Autodesk Fusion 360 part; units mm, degrees
(part 4 of 5)
  line L2596 (100.9284, -91.6876) -> (100.9149, -91.7012)
  line L2597 (100.9149, -91.7012) -> (100.9053, -91.7031)
  line L2598 (100.9053, -91.7031) -> (98.5241, -91.7031)
  line L2599 (98.5241, -91.7031) -> (98.5145, -91.7012)
  line L2600 (98.5145, -91.7012) -> (98.501, -91.6876)
  line L2601 (98.501, -91.6876) -> (98.4991, -91.6781)
  line L2602 (98.4991, -91.6781) -> (98.4991, -89.6195)
  line L2603 (98.4991, -89.6195) -> (96.1428, -89.6195)
  line L2604 (96.1428, -89.6195) -> (96.1333, -89.6176)
  line L2605 (96.1333, -89.6176) -> (96.1197, -89.6041)
  line L2606 (96.1197, -89.6041) -> (96.1178, -89.5945)
  line L2607 (96.1178, -89.5945) -> (96.1178, -86.3203)
  line L2608 (96.1178, -86.3203) -> (96.1197, -86.3107)
  line L2609 (96.1197, -86.3107) -> (96.1333, -86.2972)
  line L2610 (96.1333, -86.2972) -> (96.1428, -86.2953)
  line L2611 (96.1428, -86.2953) -> (98.4991, -86.2953)
  line L2612 (98.4991, -86.2953) -> (98.4991, -83.3437)
  line L2613 (98.4991, -83.3437) -> (98.501, -83.3341)
  line L2614 (98.501, -83.3341) -> (98.5145, -83.3206)
  line L2615 (98.5145, -83.3206) -> (98.5241, -83.3187)
  line L2616 (98.5241, -83.3187) -> (112.2163, -83.3187)
  line L2617 (112.2163, -83.3187) -> (112.2258, -83.3206)
  line L2618 (98.5491, -83.3687) -> (98.5491, -86.3203)
  line L2619 (98.5491, -86.3203) -> (98.5472, -86.3298)
  line L2620 (98.5472, -86.3298) -> (98.5336, -86.3434)
  line L2621 (98.5336, -86.3434) -> (98.5241, -86.3453)
  line L2622 (98.5241, -86.3453) -> (96.1678, -86.3453)
  line L2623 (96.1678, -86.3453) -> (96.1678, -89.5695)
  line L2624 (96.1678, -89.5695) -> (98.5241, -89.5695)
  line L2625 (98.5241, -89.5695) -> (98.5336, -89.5714)
  line L2626 (98.5336, -89.5714) -> (98.5472, -89.5849)
  line L2627 (98.5472, -89.5849) -> (98.5491, -89.5945)
  line L2628 (98.5491, -89.5945) -> (98.5491, -91.6531)
  line L2629 (98.5491, -91.6531) -> (100.8803, -91.6531)
  line L2630 (100.8803, -91.6531) -> (100.8803, -89.8921)
  line L2631 (100.8803, -89.8921) -> (100.8822, -89.8826)
  line L2632 (100.8822, -89.8826) -> (100.8958, -89.869)
  line L2633 (100.8958, -89.869) -> (100.9053, -89.8671)
  line L2634 (100.9053, -89.8671) -> (102.3936, -89.8671)
  line L2635 (102.3936, -89.8671) -> (102.4032, -89.869)
  line L2636 (102.4032, -89.869) -> (102.4167, -89.8826)
  line L2637 (102.4167, -89.8826) -> (102.4186, -89.8921)
  line L2638 (102.4186, -89.8921) -> (102.4186, -92.8437)
  line L2639 (102.4186, -92.8437) -> (102.6913, -92.8437)
  line L2640 (102.6913, -92.8437) -> (107.1311, -92.8437)
  line L2641 (107.1311, -92.8437) -> (107.1311, -91.6781)
  line L2642 (107.1311, -91.6781) -> (107.1311, -87.8086)
  line L2643 (107.1311, -87.8086) -> (107.133, -87.799)
  line L2644 (107.133, -87.799) -> (107.1465, -87.7855)
  line L2645 (107.1465, -87.7855) -> (107.1561, -87.7836)
  line L2646 (107.1561, -87.7836) -> (109.81, -87.7836)
  line L2647 (109.81, -87.7836) -> (109.81, -86.9156)
  line L2648 (109.81, -86.9156) -> (109.8119, -86.906)
  line L2649 (109.8119, -86.906) -> (109.8254, -86.8925)
  line L2650 (109.8254, -86.8925) -> (109.835, -86.8906)
  line L2651 (109.835, -86.8906) -> (112.1913, -86.8906)
  line L2652 (112.1913, -86.8906) -> (112.1913, -83.3687)
  line L2653 (112.1913, -83.3687) -> (98.5491, -83.3687)
  line L2654 (131.2758, -83.3206) -> (131.2894, -83.3341)
  line L2655 (131.2894, -83.3341) -> (131.2913, -83.3437)
  line L2656 (131.2913, -83.3437) -> (131.2913, -86.9156)
  line L2657 (131.2913, -86.9156) -> (131.2894, -86.9252)
  line L2658 (131.2894, -86.9252) -> (131.2758, -86.9387)
  line L2659 (131.2758, -86.9387) -> (131.2663, -86.9406)
  line L2660 (131.2663, -86.9406) -> (128.91, -86.9406)
  line L2661 (128.91, -86.9406) -> (128.91, -87.8086)
  line L2662 (128.91, -87.8086) -> (128.9081, -87.8181)
  line L2663 (128.9081, -87.8181) -> (128.8946, -87.8316)
  line L2664 (128.8946, -87.8316) -> (128.885, -87.8336)
  line L2665 (128.885, -87.8336) -> (126.2311, -87.8336)
  line L2666 (126.2311, -87.8336) -> (126.2311, -91.6781)
  line L2667 (126.2311, -91.6781) -> (126.2311, -92.8687)
  line L2668 (126.2311, -92.8687) -> (126.2292, -92.8783)
  line L2669 (126.2292, -92.8783) -> (126.2157, -92.8918)
  line L2670 (126.2157, -92.8918) -> (126.2061, -92.8937)
  line L2671 (126.2061, -92.8937) -> (121.7413, -92.8937)
  line L2672 (121.7413, -92.8937) -> (121.4436, -92.8937)
  line L2673 (121.4436, -92.8937) -> (121.434, -92.8918)
  line L2674 (121.434, -92.8918) -> (121.4205, -92.8783)
  line L2675 (121.4205, -92.8783) -> (121.4186, -92.8687)
  line L2676 (121.4186, -92.8687) -> (121.4186, -89.9171)
  line L2677 (121.4186, -89.9171) -> (119.9803, -89.9171)
  line L2678 (119.9803, -89.9171) -> (119.9803, -91.6781)
  line L2679 (119.9803, -91.6781) -> (119.9784, -91.6876)
  line L2680 (119.9784, -91.6876) -> (119.9649, -91.7012)
  line L2681 (119.9649, -91.7012) -> (119.9553, -91.7031)
  line L2682 (119.9553, -91.7031) -> (117.5741, -91.7031)
  line L2683 (117.5741, -91.7031) -> (117.5645, -91.7012)
  line L2684 (117.5645, -91.7012) -> (117.551, -91.6876)
  line L2685 (117.551, -91.6876) -> (117.5491, -91.6781)
  line L2686 (117.5491, -91.6781) -> (117.5491, -89.6195)
  line L2687 (117.5491, -89.6195) -> (115.1928, -89.6195)
  line L2688 (115.1928, -89.6195) -> (115.1833, -89.6176)
  line L2689 (115.1833, -89.6176) -> (115.1697, -89.6041)
  line L2690 (115.1697, -89.6041) -> (115.1678, -89.5945)
  line L2691 (115.1678, -89.5945) -> (115.1678, -86.3203)
  line L2692 (115.1678, -86.3203) -> (115.1697, -86.3107)
  line L2693 (115.1697, -86.3107) -> (115.1833, -86.2972)
  line L2694 (115.1833, -86.2972) -> (115.1928, -86.2953)
  line L2695 (115.1928, -86.2953) -> (117.5491, -86.2953)
  line L2696 (117.5491, -86.2953) -> (117.5491, -83.3437)
  line L2697 (117.5491, -83.3437) -> (117.551, -83.3341)
  line L2698 (117.551, -83.3341) -> (117.5645, -83.3206)
  line L2699 (117.5645, -83.3206) -> (117.5741, -83.3187)
  line L2700 (117.5741, -83.3187) -> (131.2663, -83.3187)
  line L2701 (131.2663, -83.3187) -> (131.2758, -83.3206)
  line L2702 (117.5991, -83.3687) -> (117.5991, -86.3203)
  line L2703 (117.5991, -86.3203) -> (117.5972, -86.3298)
  line L2704 (117.5972, -86.3298) -> (117.5836, -86.3434)
  line L2705 (117.5836, -86.3434) -> (117.5741, -86.3453)
  line L2706 (117.5741, -86.3453) -> (115.2178, -86.3453)
  line L2707 (115.2178, -86.3453) -> (115.2178, -89.5695)
  line L2708 (115.2178, -89.5695) -> (117.5741, -89.5695)
  line L2709 (117.5741, -89.5695) -> (117.5836, -89.5714)
  line L2710 (117.5836, -89.5714) -> (117.5972, -89.5849)
  line L2711 (117.5972, -89.5849) -> (117.5991, -89.5945)
  line L2712 (117.5991, -89.5945) -> (117.5991, -91.6531)
  line L2713 (117.5991, -91.6531) -> (119.9303, -91.6531)
  line L2714 (119.9303, -91.6531) -> (119.9303, -89.8921)
  line L2715 (119.9303, -89.8921) -> (119.9322, -89.8826)
  line L2716 (119.9322, -89.8826) -> (119.9458, -89.869)
  line L2717 (119.9458, -89.869) -> (119.9553, -89.8671)
  line L2718 (119.9553, -89.8671) -> (121.4436, -89.8671)
  line L2719 (121.4436, -89.8671) -> (121.4532, -89.869)
  line L2720 (121.4532, -89.869) -> (121.4667, -89.8826)
  line L2721 (121.4667, -89.8826) -> (121.4686, -89.8921)
  line L2722 (121.4686, -89.8921) -> (121.4686, -92.8437)
  line L2723 (121.4686, -92.8437) -> (121.7413, -92.8437)
  line L2724 (121.7413, -92.8437) -> (126.1811, -92.8437)
  line L2725 (126.1811, -92.8437) -> (126.1811, -91.6781)
  line L2726 (126.1811, -91.6781) -> (126.1811, -87.8086)
  line L2727 (126.1811, -87.8086) -> (126.183, -87.799)
  line L2728 (126.183, -87.799) -> (126.1965, -87.7855)
  line L2729 (126.1965, -87.7855) -> (126.2061, -87.7836)
  line L2730 (126.2061, -87.7836) -> (128.86, -87.7836)
  line L2731 (128.86, -87.7836) -> (128.86, -86.9156)
  line L2732 (128.86, -86.9156) -> (128.8619, -86.906)
  line L2733 (128.8619, -86.906) -> (128.8754, -86.8925)
  line L2734 (128.8754, -86.8925) -> (128.885, -86.8906)
  line L2735 (128.885, -86.8906) -> (131.2413, -86.8906)
  line L2736 (131.2413, -86.8906) -> (131.2413, -83.3687)
  line L2737 (131.2413, -83.3687) -> (117.5991, -83.3687)
  line L2738 (93.1758, -83.3205) -> (93.1894, -83.3341)
  line L2739 (93.1894, -83.3341) -> (93.1913, -83.3436)
  line L2740 (93.1913, -83.3436) -> (93.1913, -86.9155)
  line L2741 (93.1913, -86.9155) -> (93.1894, -86.9251)
  line L2742 (93.1894, -86.9251) -> (93.1758, -86.9386)
  line L2743 (93.1758, -86.9386) -> (93.1663, -86.9405)
  line L2744 (93.1663, -86.9405) -> (90.81, -86.9405)
  line L2745 (90.81, -86.9405) -> (90.81, -87.8085)
  line L2746 (90.81, -87.8085) -> (90.8081, -87.818)
  line L2747 (90.8081, -87.818) -> (90.7946, -87.8316)
  line L2748 (90.7946, -87.8316) -> (90.785, -87.8335)
  line L2749 (90.785, -87.8335) -> (88.1311, -87.8335)
  line L2750 (88.1311, -87.8335) -> (88.1311, -91.678)
  line L2751 (88.1311, -91.678) -> (88.1311, -92.8686)
  line L2752 (88.1311, -92.8686) -> (88.1292, -92.8782)
  line L2753 (88.1292, -92.8782) -> (88.1157, -92.8917)
  line L2754 (88.1157, -92.8917) -> (88.1061, -92.8936)
  line L2755 (88.1061, -92.8936) -> (83.6413, -92.8936)
  line L2756 (83.6413, -92.8936) -> (83.3436, -92.8936)
  line L2757 (83.3436, -92.8936) -> (83.334, -92.8917)
  line L2758 (83.334, -92.8917) -> (83.3205, -92.8782)
  line L2759 (83.3205, -92.8782) -> (83.3186, -92.8686)
  line L2760 (83.3186, -92.8686) -> (83.3186, -89.9171)
  line L2761 (83.3186, -89.9171) -> (81.8803, -89.9171)
  line L2762 (81.8803, -89.9171) -> (81.8803, -91.678)
  line L2763 (81.8803, -91.678) -> (81.8784, -91.6876)
  line L2764 (81.8784, -91.6876) -> (81.8649, -91.7011)
  line L2765 (81.8649, -91.7011) -> (81.8553, -91.703)
  line L2766 (81.8553, -91.703) -> (79.4741, -91.703)
  line L2767 (79.4741, -91.703) -> (79.4645, -91.7011)
  line L2768 (79.4645, -91.7011) -> (79.451, -91.6876)
  line L2769 (79.451, -91.6876) -> (79.4491, -91.678)
  line L2770 (79.4491, -91.678) -> (79.4491, -89.6194)
  line L2771 (79.4491, -89.6194) -> (77.0928, -89.6194)
  line L2772 (77.0928, -89.6194) -> (77.0833, -89.6175)
  line L2773 (77.0833, -89.6175) -> (77.0697, -89.604)
  line L2774 (77.0697, -89.604) -> (77.0678, -89.5944)
  line L2775 (77.0678, -89.5944) -> (77.0678, -86.3202)
  line L2776 (77.0678, -86.3202) -> (77.0697, -86.3106)
  line L2777 (77.0697, -86.3106) -> (77.0833, -86.2971)
  line L2778 (77.0833, -86.2971) -> (77.0928, -86.2952)
  line L2779 (77.0928, -86.2952) -> (79.4491, -86.2952)
  line L2780 (79.4491, -86.2952) -> (79.4491, -83.3436)
  line L2781 (79.4491, -83.3436) -> (79.451, -83.3341)
  line L2782 (79.451, -83.3341) -> (79.4645, -83.3205)
  line L2783 (79.4645, -83.3205) -> (79.4741, -83.3186)
  line L2784 (79.4741, -83.3186) -> (93.1663, -83.3186)
  line L2785 (93.1663, -83.3186) -> (93.1758, -83.3205)
  line L2786 (79.4991, -83.3686) -> (79.4991, -86.3202)
  line L2787 (79.4991, -86.3202) -> (79.4972, -86.3298)
  line L2788 (79.4972, -86.3298) -> (79.4836, -86.3433)
  line L2789 (79.4836, -86.3433) -> (79.4741, -86.3452)
  line L2790 (79.4741, -86.3452) -> (77.1178, -86.3452)
  line L2791 (77.1178, -86.3452) -> (77.1178, -89.5694)
  line L2792 (77.1178, -89.5694) -> (79.4741, -89.5694)
  line L2793 (79.4741, -89.5694) -> (79.4836, -89.5713)
  line L2794 (79.4836, -89.5713) -> (79.4972, -89.5848)
  line L2795 (79.4972, -89.5848) -> (79.4991, -89.5944)
  line L2796 (79.4991, -89.5944) -> (79.4991, -91.653)
  line L2797 (79.4991, -91.653) -> (81.8303, -91.653)
  line L2798 (81.8303, -91.653) -> (81.8303, -89.8921)
  line L2799 (81.8303, -89.8921) -> (81.8322, -89.8825)
  line L2800 (81.8322, -89.8825) -> (81.8458, -89.869)
  line L2801 (81.8458, -89.869) -> (81.8553, -89.8671)
  line L2802 (81.8553, -89.8671) -> (83.3436, -89.8671)
  line L2803 (83.3436, -89.8671) -> (83.3532, -89.869)
  line L2804 (83.3532, -89.869) -> (83.3667, -89.8825)
  line L2805 (83.3667, -89.8825) -> (83.3686, -89.8921)
  line L2806 (83.3686, -89.8921) -> (83.3686, -92.8436)
  line L2807 (83.3686, -92.8436) -> (83.6413, -92.8436)
  line L2808 (83.6413, -92.8436) -> (88.0811, -92.8436)
  line L2809 (88.0811, -92.8436) -> (88.0811, -91.678)
  line L2810 (88.0811, -91.678) -> (88.0811, -87.8085)
  line L2811 (88.0811, -87.8085) -> (88.083, -87.7989)
  line L2812 (88.083, -87.7989) -> (88.0965, -87.7854)
  line L2813 (88.0965, -87.7854) -> (88.1061, -87.7835)
  line L2814 (88.1061, -87.7835) -> (90.76, -87.7835)
  line L2815 (90.76, -87.7835) -> (90.76, -86.9155)
  line L2816 (90.76, -86.9155) -> (90.7619, -86.9059)
  line L2817 (90.7619, -86.9059) -> (90.7754, -86.8924)
  line L2818 (90.7754, -86.8924) -> (90.785, -86.8905)
  line L2819 (90.785, -86.8905) -> (93.1413, -86.8905)
  line L2820 (93.1413, -86.8905) -> (93.1413, -83.3686)
  line L2821 (93.1413, -83.3686) -> (79.4991, -83.3686)
  line L2822 (150.3258, -83.3205) -> (150.3394, -83.3341)
  line L2823 (150.3394, -83.3341) -> (150.3413, -83.3436)
  line L2824 (150.3413, -83.3436) -> (150.3413, -86.9155)
  line L2825 (150.3413, -86.9155) -> (150.3394, -86.9251)
  line L2826 (150.3394, -86.9251) -> (150.3258, -86.9386)
  line L2827 (150.3258, -86.9386) -> (150.3163, -86.9405)
  line L2828 (150.3163, -86.9405) -> (147.96, -86.9405)
  line L2829 (147.96, -86.9405) -> (147.96, -87.8085)
  line L2830 (147.96, -87.8085) -> (147.9581, -87.818)
  line L2831 (147.9581, -87.818) -> (147.9446, -87.8316)
  line L2832 (147.9446, -87.8316) -> (147.935, -87.8335)
  line L2833 (147.935, -87.8335) -> (145.2811, -87.8335)
  line L2834 (145.2811, -87.8335) -> (145.2811, -91.678)
  line L2835 (145.2811, -91.678) -> (145.2811, -92.8686)
  line L2836 (145.2811, -92.8686) -> (145.2792, -92.8782)
  line L2837 (145.2792, -92.8782) -> (145.2657, -92.8917)
  line L2838 (145.2657, -92.8917) -> (145.2561, -92.8936)
  line L2839 (145.2561, -92.8936) -> (140.7913, -92.8936)
  line L2840 (140.7913, -92.8936) -> (140.4936, -92.8936)
  line L2841 (140.4936, -92.8936) -> (140.484, -92.8917)
  line L2842 (140.484, -92.8917) -> (140.4705, -92.8782)
  line L2843 (140.4705, -92.8782) -> (140.4686, -92.8686)
  line L2844 (140.4686, -92.8686) -> (140.4686, -89.9171)
  line L2845 (140.4686, -89.9171) -> (139.0303, -89.9171)
  line L2846 (139.0303, -89.9171) -> (139.0303, -91.678)
  line L2847 (139.0303, -91.678) -> (139.0284, -91.6876)
  line L2848 (139.0284, -91.6876) -> (139.0149, -91.7011)
  line L2849 (139.0149, -91.7011) -> (139.0053, -91.703)
  line L2850 (139.0053, -91.703) -> (136.6241, -91.703)
  line L2851 (136.6241, -91.703) -> (136.6145, -91.7011)
  line L2852 (136.6145, -91.7011) -> (136.601, -91.6876)
  line L2853 (136.601, -91.6876) -> (136.5991, -91.678)
  line L2854 (136.5991, -91.678) -> (136.5991, -89.6194)
  line L2855 (136.5991, -89.6194) -> (134.2428, -89.6194)
  line L2856 (134.2428, -89.6194) -> (134.2333, -89.6175)
  line L2857 (134.2333, -89.6175) -> (134.2197, -89.604)
  line L2858 (134.2197, -89.604) -> (134.2178, -89.5944)
  line L2859 (134.2178, -89.5944) -> (134.2178, -86.3202)
  line L2860 (134.2178, -86.3202) -> (134.2197, -86.3106)
  line L2861 (134.2197, -86.3106) -> (134.2333, -86.2971)
  line L2862 (134.2333, -86.2971) -> (134.2428, -86.2952)
  line L2863 (134.2428, -86.2952) -> (136.5991, -86.2952)
  line L2864 (136.5991, -86.2952) -> (136.5991, -83.3436)
  line L2865 (136.5991, -83.3436) -> (136.601, -83.3341)
  line L2866 (136.601, -83.3341) -> (136.6145, -83.3205)
  line L2867 (136.6145, -83.3205) -> (136.6241, -83.3186)
  line L2868 (136.6241, -83.3186) -> (150.3163, -83.3186)
  line L2869 (150.3163, -83.3186) -> (150.3258, -83.3205)
  line L2870 (136.6491, -83.3686) -> (136.6491, -86.3202)
  line L2871 (136.6491, -86.3202) -> (136.6472, -86.3298)
  line L2872 (136.6472, -86.3298) -> (136.6336, -86.3433)
  line L2873 (136.6336, -86.3433) -> (136.6241, -86.3452)
  line L2874 (136.6241, -86.3452) -> (134.2678, -86.3452)
  line L2875 (134.2678, -86.3452) -> (134.2678, -89.5694)
  line L2876 (134.2678, -89.5694) -> (136.6241, -89.5694)
  line L2877 (136.6241, -89.5694) -> (136.6336, -89.5713)
  line L2878 (136.6336, -89.5713) -> (136.6472, -89.5848)
  line L2879 (136.6472, -89.5848) -> (136.6491, -89.5944)
  line L2880 (136.6491, -89.5944) -> (136.6491, -91.653)
  line L2881 (136.6491, -91.653) -> (138.9803, -91.653)
  line L2882 (138.9803, -91.653) -> (138.9803, -89.8921)
  line L2883 (138.9803, -89.8921) -> (138.9822, -89.8825)
  line L2884 (138.9822, -89.8825) -> (138.9958, -89.869)
  line L2885 (138.9958, -89.869) -> (139.0053, -89.8671)
  line L2886 (139.0053, -89.8671) -> (140.4936, -89.8671)
  line L2887 (140.4936, -89.8671) -> (140.5032, -89.869)
  line L2888 (140.5032, -89.869) -> (140.5167, -89.8825)
  line L2889 (140.5167, -89.8825) -> (140.5186, -89.8921)
  line L2890 (140.5186, -89.8921) -> (140.5186, -92.8436)
  line L2891 (140.5186, -92.8436) -> (140.7913, -92.8436)
  line L2892 (140.7913, -92.8436) -> (145.2311, -92.8436)
  line L2893 (145.2311, -92.8436) -> (145.2311, -91.678)
  line L2894 (145.2311, -91.678) -> (145.2311, -87.8085)
  line L2895 (145.2311, -87.8085) -> (145.233, -87.7989)
  line L2896 (145.233, -87.7989) -> (145.2465, -87.7854)
  line L2897 (145.2465, -87.7854) -> (145.2561, -87.7835)
  line L2898 (145.2561, -87.7835) -> (147.91, -87.7835)
  line L2899 (147.91, -87.7835) -> (147.91, -86.9155)
  line L2900 (147.91, -86.9155) -> (147.9119, -86.9059)
  line L2901 (147.9119, -86.9059) -> (147.9254, -86.8924)
  line L2902 (147.9254, -86.8924) -> (147.935, -86.8905)
  line L2903 (147.935, -86.8905) -> (150.2913, -86.8905)
  line L2904 (150.2913, -86.8905) -> (150.2913, -83.3686)
  line L2905 (150.2913, -83.3686) -> (136.6491, -83.3686)
  line L2906 (110.0461, -89.2903) -> (110.2508, -89.3451)
  line L2907 (110.2508, -89.3451) -> (110.4428, -89.4347)
  line L2908 (110.4428, -89.4347) -> (110.6164, -89.5562)
  line L2909 (110.6164, -89.5562) -> (110.7662, -89.7061)
  line L2910 (110.7662, -89.7061) -> (110.8878, -89.8796)
  line L2911 (110.8878, -89.8796) -> (110.9773, -90.0717)
  line L2912 (110.9773, -90.0717) -> (111.0322, -90.2764)
  line L2913 (111.0322, -90.2764) -> (111.0506, -90.4875)
  line L2914 (111.0506, -90.4875) -> (111.0322, -90.6985)
  line L2915 (111.0322, -90.6985) -> (110.9773, -90.9032)
  line L2916 (110.9773, -90.9032) -> (110.8878, -91.0953)
  line L2917 (110.8878, -91.0953) -> (110.7662, -91.2688)
  line L2918 (110.7662, -91.2688) -> (110.6164, -91.4187)
  line L2919 (110.6164, -91.4187) -> (110.4428, -91.5402)
  line L2920 (110.4428, -91.5402) -> (110.2508, -91.6298)
  line L2921 (110.2508, -91.6298) -> (110.0461, -91.6846)
  line L2922 (110.0461, -91.6846) -> (109.835, -91.7031)
  line L2923 (109.835, -91.7031) -> (109.6239, -91.6846)
  line L2924 (109.6239, -91.6846) -> (109.4192, -91.6298)
  line L2925 (109.4192, -91.6298) -> (109.2272, -91.5402)
  line L2926 (109.2272, -91.5402) -> (109.0536, -91.4187)
  line L2927 (109.0536, -91.4187) -> (108.9038, -91.2688)
  line L2928 (108.9038, -91.2688) -> (108.7822, -91.0953)
  line L2929 (108.7822, -91.0953) -> (108.6927, -90.9032)
  line L2930 (108.6927, -90.9032) -> (108.6379, -90.6985)
  line L2931 (108.6379, -90.6985) -> (108.6194, -90.4875)
  line L2932 (108.6194, -90.4875) -> (108.6379, -90.2764)
  line L2933 (108.6379, -90.2764) -> (108.6927, -90.0717)
  line L2934 (108.6927, -90.0717) -> (108.7822, -89.8796)
  line L2935 (108.7822, -89.8796) -> (108.9038, -89.7061)
  line L2936 (108.9038, -89.7061) -> (109.0536, -89.5562)
  line L2937 (109.0536, -89.5562) -> (109.2272, -89.4347)
  line L2938 (109.2272, -89.4347) -> (109.4192, -89.3451)
  line L2939 (109.4192, -89.3451) -> (109.6239, -89.2903)
  line L2940 (109.6239, -89.2903) -> (109.835, -89.2718)
  line L2941 (109.835, -89.2718) -> (110.0461, -89.2903)
  line L2942 (108.6843, -90.7026) -> (108.7434, -90.9103)
  line L2943 (108.7434, -90.9103) -> (108.8397, -91.1037)
  line L2944 (108.8397, -91.1037) -> (108.9699, -91.2761)
  line L2945 (108.9699, -91.2761) -> (109.1296, -91.4216)
  line L2946 (109.1296, -91.4216) -> (109.3132, -91.5353)
  line L2947 (109.3132, -91.5353) -> (109.5147, -91.6134)
  line L2948 (109.5147, -91.6134) -> (109.727, -91.6531)
  line L2949 (109.727, -91.6531) -> (109.943, -91.6531)
  line L2950 (109.943, -91.6531) -> (110.1554, -91.6134)
  line L2951 (110.1554, -91.6134) -> (110.3568, -91.5353)
  line L2952 (110.3568, -91.5353) -> (110.5405, -91.4216)
  line L2953 (110.5405, -91.4216) -> (110.7001, -91.2761)
  line L2954 (110.7001, -91.2761) -> (110.8303, -91.1037)
  line L2955 (110.8303, -91.1037) -> (110.9266, -90.9103)
  line L2956 (110.9266, -90.9103) -> (110.9857, -90.7026)
  line L2957 (110.9857, -90.7026) -> (111.0056, -90.4875)
  line L2958 (111.0056, -90.4875) -> (110.9857, -90.2724)
  line L2959 (110.9857, -90.2724) -> (110.9266, -90.0646)
  line L2960 (110.9266, -90.0646) -> (110.8303, -89.8712)
  line L2961 (110.8303, -89.8712) -> (110.7001, -89.6988)
  line L2962 (110.7001, -89.6988) -> (110.5405, -89.5533)
  line L2963 (110.5405, -89.5533) -> (110.3568, -89.4396)
  line L2964 (110.3568, -89.4396) -> (110.1554, -89.3615)
  line L2965 (110.1554, -89.3615) -> (109.943, -89.3218)
  line L2966 (109.943, -89.3218) -> (109.727, -89.3218)
  line L2967 (109.727, -89.3218) -> (109.5147, -89.3615)
  line L2968 (109.5147, -89.3615) -> (109.3132, -89.4396)
  line L2969 (109.3132, -89.4396) -> (109.1296, -89.5533)
  line L2970 (109.1296, -89.5533) -> (108.9699, -89.6988)
  line L2971 (108.9699, -89.6988) -> (108.8397, -89.8712)
  line L2972 (108.8397, -89.8712) -> (108.7434, -90.0646)
  line L2973 (108.7434, -90.0646) -> (108.6843, -90.2724)
  line L2974 (108.6843, -90.2724) -> (108.6644, -90.4875)
  line L2975 (108.6644, -90.4875) -> (108.6843, -90.7026)
  line L2976 (129.0961, -89.2903) -> (129.3008, -89.3451)
  line L2977 (129.3008, -89.3451) -> (129.4928, -89.4347)
  line L2978 (129.4928, -89.4347) -> (129.6664, -89.5562)
  line L2979 (129.6664, -89.5562) -> (129.8162, -89.7061)
  line L2980 (129.8162, -89.7061) -> (129.9378, -89.8796)
  line L2981 (129.9378, -89.8796) -> (130.0273, -90.0717)
  line L2982 (130.0273, -90.0717) -> (130.0822, -90.2764)
  line L2983 (130.0822, -90.2764) -> (130.1006, -90.4875)
  line L2984 (130.1006, -90.4875) -> (130.0822, -90.6985)
  line L2985 (130.0822, -90.6985) -> (130.0273, -90.9032)
  line L2986 (130.0273, -90.9032) -> (129.9378, -91.0953)
  line L2987 (129.9378, -91.0953) -> (129.8162, -91.2688)
  line L2988 (129.8162, -91.2688) -> (129.6664, -91.4187)
  line L2989 (129.6664, -91.4187) -> (129.4928, -91.5402)
  line L2990 (129.4928, -91.5402) -> (129.3008, -91.6298)
  line L2991 (129.3008, -91.6298) -> (129.0961, -91.6846)
  line L2992 (129.0961, -91.6846) -> (128.885, -91.7031)
  line L2993 (128.885, -91.7031) -> (128.6739, -91.6846)
  line L2994 (128.6739, -91.6846) -> (128.4692, -91.6298)
  line L2995 (128.4692, -91.6298) -> (128.2772, -91.5402)
  line L2996 (128.2772, -91.5402) -> (128.1036, -91.4187)
  line L2997 (128.1036, -91.4187) -> (127.9538, -91.2688)
  line L2998 (127.9538, -91.2688) -> (127.8322, -91.0953)
  line L2999 (127.8322, -91.0953) -> (127.7427, -90.9032)
  line L3000 (127.7427, -90.9032) -> (127.6879, -90.6985)
  line L3001 (127.6879, -90.6985) -> (127.6694, -90.4875)
  line L3002 (127.6694, -90.4875) -> (127.6879, -90.2764)
  line L3003 (127.6879, -90.2764) -> (127.7427, -90.0717)
  line L3004 (127.7427, -90.0717) -> (127.8322, -89.8796)
  line L3005 (127.8322, -89.8796) -> (127.9538, -89.7061)
  line L3006 (127.9538, -89.7061) -> (128.1036, -89.5562)
  line L3007 (128.1036, -89.5562) -> (128.2772, -89.4347)
  line L3008 (128.2772, -89.4347) -> (128.4692, -89.3451)
  line L3009 (128.4692, -89.3451) -> (128.6739, -89.2903)
  line L3010 (128.6739, -89.2903) -> (128.885, -89.2718)
  line L3011 (128.885, -89.2718) -> (129.0961, -89.2903)
  line L3012 (127.7343, -90.7026) -> (127.7934, -90.9103)
  line L3013 (127.7934, -90.9103) -> (127.8897, -91.1037)
  line L3014 (127.8897, -91.1037) -> (128.0199, -91.2761)
  line L3015 (128.0199, -91.2761) -> (128.1796, -91.4216)
  line L3016 (128.1796, -91.4216) -> (128.3632, -91.5353)
  line L3017 (128.3632, -91.5353) -> (128.5647, -91.6134)
  line L3018 (128.5647, -91.6134) -> (128.777, -91.6531)
  line L3019 (128.777, -91.6531) -> (128.993, -91.6531)
  line L3020 (128.993, -91.6531) -> (129.2054, -91.6134)
  line L3021 (129.2054, -91.6134) -> (129.4068, -91.5353)
  line L3022 (129.4068, -91.5353) -> (129.5905, -91.4216)
  line L3023 (129.5905, -91.4216) -> (129.7501, -91.2761)
  line L3024 (129.7501, -91.2761) -> (129.8803, -91.1037)
  line L3025 (129.8803, -91.1037) -> (129.9766, -90.9103)
  line L3026 (129.9766, -90.9103) -> (130.0357, -90.7026)
  line L3027 (130.0357, -90.7026) -> (130.0556, -90.4875)
  line L3028 (130.0556, -90.4875) -> (130.0357, -90.2724)
  line L3029 (130.0357, -90.2724) -> (129.9766, -90.0646)
  line L3030 (129.9766, -90.0646) -> (129.8803, -89.8712)
  line L3031 (129.8803, -89.8712) -> (129.7501, -89.6988)
  line L3032 (129.7501, -89.6988) -> (129.5905, -89.5533)
  line L3033 (129.5905, -89.5533) -> (129.4068, -89.4396)
  line L3034 (129.4068, -89.4396) -> (129.2054, -89.3615)
  line L3035 (129.2054, -89.3615) -> (128.993, -89.3218)
  line L3036 (128.993, -89.3218) -> (128.777, -89.3218)
  line L3037 (128.777, -89.3218) -> (128.5647, -89.3615)
  line L3038 (128.5647, -89.3615) -> (128.3632, -89.4396)
  line L3039 (128.3632, -89.4396) -> (128.1796, -89.5533)
  line L3040 (128.1796, -89.5533) -> (128.0199, -89.6988)
  line L3041 (128.0199, -89.6988) -> (127.8897, -89.8712)
  line L3042 (127.8897, -89.8712) -> (127.7934, -90.0646)
  line L3043 (127.7934, -90.0646) -> (127.7343, -90.2724)
  line L3044 (127.7343, -90.2724) -> (127.7144, -90.4875)
  line L3045 (127.7144, -90.4875) -> (127.7343, -90.7026)
  line L3046 (90.9961, -89.2902) -> (91.2008, -89.3451)
  line L3047 (91.2008, -89.3451) -> (91.3928, -89.4346)
  line L3048 (91.3928, -89.4346) -> (91.5664, -89.5562)
  line L3049 (91.5664, -89.5562) -> (91.7162, -89.706)
  line L3050 (91.7162, -89.706) -> (91.8378, -89.8796)
  line L3051 (91.8378, -89.8796) -> (91.9273, -90.0716)
  line L3052 (91.9273, -90.0716) -> (91.9822, -90.2763)
  line L3053 (91.9822, -90.2763) -> (92.0006, -90.4874)
  line L3054 (92.0006, -90.4874) -> (91.9822, -90.6985)
  line L3055 (91.9822, -90.6985) -> (91.9273, -90.9031)
  line L3056 (91.9273, -90.9031) -> (91.8378, -91.0952)
  line L3057 (91.8378, -91.0952) -> (91.7162, -91.2688)
  line L3058 (91.7162, -91.2688) -> (91.5664, -91.4186)
  line L3059 (91.5664, -91.4186) -> (91.3928, -91.5401)
  line L3060 (91.3928, -91.5401) -> (91.2008, -91.6297)
  line L3061 (91.2008, -91.6297) -> (90.9961, -91.6845)
  line L3062 (90.9961, -91.6845) -> (90.785, -91.703)
  line L3063 (90.785, -91.703) -> (90.5739, -91.6845)
  line L3064 (90.5739, -91.6845) -> (90.3692, -91.6297)
  line L3065 (90.3692, -91.6297) -> (90.1772, -91.5401)
  line L3066 (90.1772, -91.5401) -> (90.0036, -91.4186)
  line L3067 (90.0036, -91.4186) -> (89.8538, -91.2688)
  line L3068 (89.8538, -91.2688) -> (89.7322, -91.0952)
  line L3069 (89.7322, -91.0952) -> (89.6427, -90.9031)
  line L3070 (89.6427, -90.9031) -> (89.5879, -90.6985)
  line L3071 (89.5879, -90.6985) -> (89.5694, -90.4874)
  line L3072 (89.5694, -90.4874) -> (89.5879, -90.2763)
  line L3073 (89.5879, -90.2763) -> (89.6427, -90.0716)
  line L3074 (89.6427, -90.0716) -> (89.7322, -89.8796)
  line L3075 (89.7322, -89.8796) -> (89.8538, -89.706)
  line L3076 (89.8538, -89.706) -> (90.0036, -89.5562)
  line L3077 (90.0036, -89.5562) -> (90.1772, -89.4346)
  line L3078 (90.1772, -89.4346) -> (90.3692, -89.3451)
  line L3079 (90.3692, -89.3451) -> (90.5739, -89.2902)
  line L3080 (90.5739, -89.2902) -> (90.785, -89.2718)
  line L3081 (90.785, -89.2718) -> (90.9961, -89.2902)
  line L3082 (89.6343, -90.7025) -> (89.6934, -90.9103)
  line L3083 (89.6934, -90.9103) -> (89.7897, -91.1036)
  line L3084 (89.7897, -91.1036) -> (89.9199, -91.276)
  line L3085 (89.9199, -91.276) -> (90.0796, -91.4215)
  line L3086 (90.0796, -91.4215) -> (90.2632, -91.5353)
  line L3087 (90.2632, -91.5353) -> (90.4647, -91.6133)
  line L3088 (90.4647, -91.6133) -> (90.677, -91.653)
  line L3089 (90.677, -91.653) -> (90.893, -91.653)
  line L3090 (90.893, -91.653) -> (91.1054, -91.6133)
  line L3091 (91.1054, -91.6133) -> (91.3068, -91.5353)
  line L3092 (91.3068, -91.5353) -> (91.4905, -91.4215)
  line L3093 (91.4905, -91.4215) -> (91.6501, -91.276)
  line L3094 (91.6501, -91.276) -> (91.7803, -91.1036)
  line L3095 (91.7803, -91.1036) -> (91.8766, -90.9103)
  line L3096 (91.8766, -90.9103) -> (91.9357, -90.7025)
  line L3097 (91.9357, -90.7025) -> (91.9556, -90.4874)
  line L3098 (91.9556, -90.4874) -> (91.9357, -90.2723)
  line L3099 (91.9357, -90.2723) -> (91.8766, -90.0645)
  line L3100 (91.8766, -90.0645) -> (91.7803, -89.8711)
  line L3101 (91.7803, -89.8711) -> (91.6501, -89.6987)
  line L3102 (91.6501, -89.6987) -> (91.4905, -89.5532)
  line L3103 (91.4905, -89.5532) -> (91.3068, -89.4395)
  line L3104 (91.3068, -89.4395) -> (91.1054, -89.3614)
  line L3105 (91.1054, -89.3614) -> (90.893, -89.3218)
  line L3106 (90.893, -89.3218) -> (90.677, -89.3218)
  line L3107 (90.677, -89.3218) -> (90.4647, -89.3614)
  line L3108 (90.4647, -89.3614) -> (90.2632, -89.4395)
  line L3109 (90.2632, -89.4395) -> (90.0796, -89.5532)
  line L3110 (90.0796, -89.5532) -> (89.9199, -89.6987)
  line L3111 (89.9199, -89.6987) -> (89.7897, -89.8711)
  line L3112 (89.7897, -89.8711) -> (89.6934, -90.0645)
  line L3113 (89.6934, -90.0645) -> (89.6343, -90.2723)
  line L3114 (89.6343, -90.2723) -> (89.6144, -90.4874)
  line L3115 (89.6144, -90.4874) -> (89.6343, -90.7025)
  line L3116 (148.1461, -89.2902) -> (148.3508, -89.3451)
  line L3117 (148.3508, -89.3451) -> (148.5428, -89.4346)
  line L3118 (148.5428, -89.4346) -> (148.7164, -89.5562)
  line L3119 (148.7164, -89.5562) -> (148.8662, -89.706)
  line L3120 (148.8662, -89.706) -> (148.9878, -89.8796)
  line L3121 (148.9878, -89.8796) -> (149.0773, -90.0716)
  line L3122 (149.0773, -90.0716) -> (149.1322, -90.2763)
  line L3123 (149.1322, -90.2763) -> (149.1506, -90.4874)
  line L3124 (149.1506, -90.4874) -> (149.1322, -90.6985)
  line L3125 (149.1322, -90.6985) -> (149.0773, -90.9031)
  line L3126 (149.0773, -90.9031) -> (148.9878, -91.0952)
  line L3127 (148.9878, -91.0952) -> (148.8662, -91.2688)
  line L3128 (148.8662, -91.2688) -> (148.7164, -91.4186)
  line L3129 (148.7164, -91.4186) -> (148.5428, -91.5401)
  line L3130 (148.5428, -91.5401) -> (148.3508, -91.6297)
  line L3131 (148.3508, -91.6297) -> (148.1461, -91.6845)
  line L3132 (148.1461, -91.6845) -> (147.935, -91.703)
  line L3133 (147.935, -91.703) -> (147.7239, -91.6845)
  line L3134 (147.7239, -91.6845) -> (147.5192, -91.6297)
  line L3135 (147.5192, -91.6297) -> (147.3272, -91.5401)
  line L3136 (147.3272, -91.5401) -> (147.1536, -91.4186)
  line L3137 (147.1536, -91.4186) -> (147.0038, -91.2688)
  line L3138 (147.0038, -91.2688) -> (146.8822, -91.0952)
  line L3139 (146.8822, -91.0952) -> (146.7927, -90.9031)
  line L3140 (146.7927, -90.9031) -> (146.7379, -90.6985)
  line L3141 (146.7379, -90.6985) -> (146.7194, -90.4874)
  line L3142 (146.7194, -90.4874) -> (146.7379, -90.2763)
  line L3143 (146.7379, -90.2763) -> (146.7927, -90.0716)
  line L3144 (146.7927, -90.0716) -> (146.8822, -89.8796)
  line L3145 (146.8822, -89.8796) -> (147.0038, -89.706)
  line L3146 (147.0038, -89.706) -> (147.1536, -89.5562)
  line L3147 (147.1536, -89.5562) -> (147.3272, -89.4346)
  line L3148 (147.3272, -89.4346) -> (147.5192, -89.3451)
  line L3149 (147.5192, -89.3451) -> (147.7239, -89.2902)
  line L3150 (147.7239, -89.2902) -> (147.935, -89.2718)
  line L3151 (147.935, -89.2718) -> (148.1461, -89.2902)
  line L3152 (146.7843, -90.7025) -> (146.8434, -90.9103)
  line L3153 (146.8434, -90.9103) -> (146.9397, -91.1036)
  line L3154 (146.9397, -91.1036) -> (147.0699, -91.276)
  line L3155 (147.0699, -91.276) -> (147.2296, -91.4215)
  line L3156 (147.2296, -91.4215) -> (147.4132, -91.5353)
  line L3157 (147.4132, -91.5353) -> (147.6147, -91.6133)
  line L3158 (147.6147, -91.6133) -> (147.827, -91.653)
  line L3159 (147.827, -91.653) -> (148.043, -91.653)
  line L3160 (148.043, -91.653) -> (148.2554, -91.6133)
  line L3161 (148.2554, -91.6133) -> (148.4568, -91.5353)
  line L3162 (148.4568, -91.5353) -> (148.6405, -91.4215)
  line L3163 (148.6405, -91.4215) -> (148.8001, -91.276)
  line L3164 (148.8001, -91.276) -> (148.9303, -91.1036)
  line L3165 (148.9303, -91.1036) -> (149.0266, -90.9103)
  line L3166 (149.0266, -90.9103) -> (149.0857, -90.7025)
  line L3167 (149.0857, -90.7025) -> (149.1056, -90.4874)
  line L3168 (149.1056, -90.4874) -> (149.0857, -90.2723)
  line L3169 (149.0857, -90.2723) -> (149.0266, -90.0645)
  line L3170 (149.0266, -90.0645) -> (148.9303, -89.8711)
  line L3171 (148.9303, -89.8711) -> (148.8001, -89.6987)
  line L3172 (148.8001, -89.6987) -> (148.6405, -89.5532)
  line L3173 (148.6405, -89.5532) -> (148.4568, -89.4395)
  line L3174 (148.4568, -89.4395) -> (148.2554, -89.3614)
  line L3175 (148.2554, -89.3614) -> (148.043, -89.3218)
  line L3176 (148.043, -89.3218) -> (147.827, -89.3218)
  line L3177 (147.827, -89.3218) -> (147.6147, -89.3614)
  line L3178 (147.6147, -89.3614) -> (147.4132, -89.4395)
  line L3179 (147.4132, -89.4395) -> (147.2296, -89.5532)
  line L3180 (147.2296, -89.5532) -> (147.0699, -89.6987)
  line L3181 (147.0699, -89.6987) -> (146.9397, -89.8711)
  line L3182 (146.9397, -89.8711) -> (146.8434, -90.0645)
  line L3183 (146.8434, -90.0645) -> (146.7843, -90.2723)
  line L3184 (146.7843, -90.2723) -> (146.7644, -90.4874)
  line L3185 (146.7644, -90.4874) -> (146.7843, -90.7025)
  line L3186 (88.4346, -75.427) -> (88.4482, -75.4405)
  line L3187 (88.4482, -75.4405) -> (88.4501, -75.4501)
  line L3188 (88.4501, -75.4501) -> (88.4501, -76.9501)
  line L3189 (88.4501, -76.9501) -> (88.4482, -76.9596)
  line L3190 (88.4482, -76.9596) -> (88.4346, -76.9732)
  line L3191 (88.4346, -76.9732) -> (88.4251, -76.9751)
  line L3192 (88.4251, -76.9751) -> (83.0251, -76.9751)
  line L3193 (83.0251, -76.9751) -> (83.0155, -76.9732)
  line L3194 (83.0155, -76.9732) -> (83.002, -76.9596)
  line L3195 (83.002, -76.9596) -> (83.0001, -76.9501)
  line L3196 (83.0001, -76.9501) -> (83.0001, -75.4501)
  line L3197 (83.0001, -75.4501) -> (83.002, -75.4405)
  line L3198 (83.002, -75.4405) -> (83.0155, -75.427)
  line L3199 (83.0155, -75.427) -> (83.0251, -75.4251)
  line L3200 (83.0251, -75.4251) -> (88.4251, -75.4251)
  line L3201 (88.4251, -75.4251) -> (88.4346, -75.427)
  line L3202 (83.0501, -75.4751) -> (83.0501, -76.9251)
  line L3203 (83.0501, -76.9251) -> (88.4001, -76.9251)
  line L3204 (88.4001, -76.9251) -> (88.4001, -75.4751)
  line L3205 (88.4001, -75.4751) -> (83.0501, -75.4751)
  line L3206 (107.4846, -75.427) -> (107.4982, -75.4405)
  line L3207 (107.4982, -75.4405) -> (107.5001, -75.4501)
  line L3208 (107.5001, -75.4501) -> (107.5001, -76.9501)
  line L3209 (107.5001, -76.9501) -> (107.4982, -76.9596)
  line L3210 (107.4982, -76.9596) -> (107.4846, -76.9732)
  line L3211 (107.4846, -76.9732) -> (107.4751, -76.9751)
  line L3212 (107.4751, -76.9751) -> (102.0751, -76.9751)
  line L3213 (102.0751, -76.9751) -> (102.0655, -76.9732)
  line L3214 (102.0655, -76.9732) -> (102.052, -76.9596)
  line L3215 (102.052, -76.9596) -> (102.0501, -76.9501)
  line L3216 (102.0501, -76.9501) -> (102.0501, -75.4501)
  line L3217 (102.0501, -75.4501) -> (102.052, -75.4405)
  line L3218 (102.052, -75.4405) -> (102.0655, -75.427)
  line L3219 (102.0655, -75.427) -> (102.0751, -75.4251)
  line L3220 (102.0751, -75.4251) -> (107.4751, -75.4251)
  line L3221 (107.4751, -75.4251) -> (107.4846, -75.427)
  line L3222 (102.1001, -75.4751) -> (102.1001, -76.9251)
  line L3223 (102.1001, -76.9251) -> (107.4501, -76.9251)
  line L3224 (107.4501, -76.9251) -> (107.4501, -75.4751)
  line L3225 (107.4501, -75.4751) -> (102.1001, -75.4751)
  line L3226 (126.5346, -75.4269) -> (126.5481, -75.4404)
  line L3227 (126.5481, -75.4404) -> (126.55, -75.45)
  line L3228 (126.55, -75.45) -> (126.55, -76.95)
  line L3229 (126.55, -76.95) -> (126.5481, -76.9596)
  line L3230 (126.5481, -76.9596) -> (126.5346, -76.9731)
  line L3231 (126.5346, -76.9731) -> (126.525, -76.975)
  line L3232 (126.525, -76.975) -> (121.125, -76.975)
  line L3233 (121.125, -76.975) -> (121.1154, -76.9731)
  line L3234 (121.1154, -76.9731) -> (121.1019, -76.9596)
  line L3235 (121.1019, -76.9596) -> (121.1, -76.95)
  line L3236 (121.1, -76.95) -> (121.1, -75.45)
  line L3237 (121.1, -75.45) -> (121.1019, -75.4404)
  line L3238 (121.1019, -75.4404) -> (121.1154, -75.4269)
  line L3239 (121.1154, -75.4269) -> (121.125, -75.425)
  line L3240 (121.125, -75.425) -> (126.525, -75.425)
  line L3241 (126.525, -75.425) -> (126.5346, -75.4269)
  line L3242 (121.15, -75.475) -> (121.15, -76.925)
  line L3243 (121.15, -76.925) -> (126.5, -76.925)
  line L3244 (126.5, -76.925) -> (126.5, -75.475)
  line L3245 (126.5, -75.475) -> (121.15, -75.475)
  line L3246 (145.5846, -75.4269) -> (145.5981, -75.4404)
  line L3247 (145.5981, -75.4404) -> (145.6, -75.45)
  line L3248 (145.6, -75.45) -> (145.6, -76.95)
  line L3249 (145.6, -76.95) -> (145.5981, -76.9596)
  line L3250 (145.5981, -76.9596) -> (145.5846, -76.9731)
  line L3251 (145.5846, -76.9731) -> (145.575, -76.975)
  line L3252 (145.575, -76.975) -> (140.175, -76.975)
  line L3253 (140.175, -76.975) -> (140.1654, -76.9731)
  line L3254 (140.1654, -76.9731) -> (140.1519, -76.9596)
  line L3255 (140.1519, -76.9596) -> (140.15, -76.95)
  line L3256 (140.15, -76.95) -> (140.15, -75.45)
  line L3257 (140.15, -75.45) -> (140.1519, -75.4404)
  line L3258 (140.1519, -75.4404) -> (140.1654, -75.4269)
  line L3259 (140.1654, -75.4269) -> (140.175, -75.425)
  line L3260 (140.175, -75.425) -> (145.575, -75.425)
  line L3261 (145.575, -75.425) -> (145.5846, -75.4269)
  line L3262 (140.2, -75.475) -> (140.2, -76.925)
  line L3263 (140.2, -76.925) -> (145.55, -76.925)
  line L3264 (145.55, -76.925) -> (145.55, -75.475)
  line L3265 (145.55, -75.475) -> (140.2, -75.475)
  line L3266 (93.1759, -64.2706) -> (93.1894, -64.2841)
  line L3267 (93.1894, -64.2841) -> (93.1913, -64.2937)
  line L3268 (93.1913, -64.2937) -> (93.1913, -67.8656)
  line L3269 (93.1913, -67.8656) -> (93.1894, -67.8751)
  line L3270 (93.1894, -67.8751) -> (93.1759, -67.8887)
  line L3271 (93.1759, -67.8887) -> (93.1663, -67.8906)
  line L3272 (93.1663, -67.8906) -> (90.8101, -67.8906)
  line L3273 (90.8101, -67.8906) -> (90.8101, -68.7585)
  line L3274 (90.8101, -68.7585) -> (90.8082, -68.7681)
  line L3275 (90.8082, -68.7681) -> (90.7946, -68.7816)
  line L3276 (90.7946, -68.7816) -> (90.7851, -68.7835)
  line L3277 (90.7851, -68.7835) -> (88.1312, -68.7835)
  line L3278 (88.1312, -68.7835) -> (88.1312, -72.6281)
  line L3279 (88.1312, -72.6281) -> (88.1312, -73.8187)
  line L3280 (88.1312, -73.8187) -> (88.1293, -73.8283)
  line L3281 (88.1293, -73.8283) -> (88.1157, -73.8418)
  line L3282 (88.1157, -73.8418) -> (88.1062, -73.8437)
  line L3283 (88.1062, -73.8437) -> (83.6413, -73.8437)
  line L3284 (83.6413, -73.8437) -> (83.3437, -73.8437)
  line L3285 (83.3437, -73.8437) -> (83.3341, -73.8418)
  line L3286 (83.3341, -73.8418) -> (83.3206, -73.8283)
  line L3287 (83.3206, -73.8283) -> (83.3187, -73.8187)
  line L3288 (83.3187, -73.8187) -> (83.3187, -70.8671)
  line L3289 (83.3187, -70.8671) -> (81.8804, -70.8671)
  line L3290 (81.8804, -70.8671) -> (81.8804, -72.6281)
  line L3291 (81.8804, -72.6281) -> (81.8785, -72.6376)
  line L3292 (81.8785, -72.6376) -> (81.865, -72.6512)
  line L3293 (81.865, -72.6512) -> (81.8554, -72.6531)
  line L3294 (81.8554, -72.6531) -> (79.4742, -72.6531)
  line L3295 (79.4742, -72.6531) -> (79.4646, -72.6512)
  line L3296 (79.4646, -72.6512) -> (79.4511, -72.6376)
  line L3297 (79.4511, -72.6376) -> (79.4492, -72.6281)
  line L3298 (79.4492, -72.6281) -> (79.4492, -70.5695)
  line L3299 (79.4492, -70.5695) -> (77.0929, -70.5695)
  line L3300 (77.0929, -70.5695) -> (77.0833, -70.5676)
  line L3301 (77.0833, -70.5676) -> (77.0698, -70.554)
  line L3302 (77.0698, -70.554) -> (77.0679, -70.5445)
  line L3303 (77.0679, -70.5445) -> (77.0679, -67.2703)
  line L3304 (77.0679, -67.2703) -> (77.0698, -67.2607)
  line L3305 (77.0698, -67.2607) -> (77.0833, -67.2472)
  line L3306 (77.0833, -67.2472) -> (77.0929, -67.2453)
  line L3307 (77.0929, -67.2453) -> (79.4492, -67.2453)
  line L3308 (79.4492, -67.2453) -> (79.4492, -64.2937)
  line L3309 (79.4492, -64.2937) -> (79.4511, -64.2841)
  line L3310 (79.4511, -64.2841) -> (79.4646, -64.2706)
  line L3311 (79.4646, -64.2706) -> (79.4742, -64.2687)
  line L3312 (79.4742, -64.2687) -> (93.1663, -64.2687)
  line L3313 (93.1663, -64.2687) -> (93.1759, -64.2706)
  line L3314 (79.4992, -64.3187) -> (79.4992, -67.2703)
  line L3315 (79.4992, -67.2703) -> (79.4972, -67.2798)
  line L3316 (79.4972, -67.2798) -> (79.4837, -67.2934)
  line L3317 (79.4837, -67.2934) -> (79.4742, -67.2953)
  line L3318 (79.4742, -67.2953) -> (77.1179, -67.2953)
  line L3319 (77.1179, -67.2953) -> (77.1179, -70.5195)
  line L3320 (77.1179, -70.5195) -> (79.4742, -70.5195)
  line L3321 (79.4742, -70.5195) -> (79.4837, -70.5214)
  line L3322 (79.4837, -70.5214) -> (79.4972, -70.5349)
  line L3323 (79.4972, -70.5349) -> (79.4992, -70.5445)
  line L3324 (79.4992, -70.5445) -> (79.4992, -72.6031)
  line L3325 (79.4992, -72.6031) -> (81.8304, -72.6031)
  line L3326 (81.8304, -72.6031) -> (81.8304, -70.8421)
  line L3327 (81.8304, -70.8421) -> (81.8323, -70.8326)
  line L3328 (81.8323, -70.8326) -> (81.8458, -70.819)
  line L3329 (81.8458, -70.819) -> (81.8554, -70.8171)
  line L3330 (81.8554, -70.8171) -> (83.3437, -70.8171)
  line L3331 (83.3437, -70.8171) -> (83.3532, -70.819)
  line L3332 (83.3532, -70.819) -> (83.3668, -70.8326)
  line L3333 (83.3668, -70.8326) -> (83.3687, -70.8421)
  line L3334 (83.3687, -70.8421) -> (83.3687, -73.7937)
  line L3335 (83.3687, -73.7937) -> (83.6413, -73.7937)
  line L3336 (83.6413, -73.7937) -> (88.0812, -73.7937)
  line L3337 (88.0812, -73.7937) -> (88.0812, -72.6281)
  line L3338 (88.0812, -72.6281) -> (88.0812, -68.7585)
  line L3339 (88.0812, -68.7585) -> (88.0831, -68.749)
  line L3340 (88.0831, -68.749) -> (88.0966, -68.7354)
  line L3341 (88.0966, -68.7354) -> (88.1062, -68.7335)
  line L3342 (88.1062, -68.7335) -> (90.7601, -68.7335)
  line L3343 (90.7601, -68.7335) -> (90.7601, -67.8656)
  line L3344 (90.7601, -67.8656) -> (90.762, -67.856)
  line L3345 (90.762, -67.856) -> (90.7755, -67.8425)
  line L3346 (90.7755, -67.8425) -> (90.7851, -67.8406)
  line L3347 (90.7851, -67.8406) -> (93.1413, -67.8406)
  line L3348 (93.1413, -67.8406) -> (93.1413, -64.3187)
  line L3349 (93.1413, -64.3187) -> (79.4992, -64.3187)
  line L3350 (112.2259, -64.2706) -> (112.2394, -64.2841)
  line L3351 (112.2394, -64.2841) -> (112.2413, -64.2937)
  line L3352 (112.2413, -64.2937) -> (112.2413, -67.8656)
  line L3353 (112.2413, -67.8656) -> (112.2394, -67.8751)
  line L3354 (112.2394, -67.8751) -> (112.2259, -67.8887)
  line L3355 (112.2259, -67.8887) -> (112.2163, -67.8906)
  line L3356 (112.2163, -67.8906) -> (109.8601, -67.8906)
  line L3357 (109.8601, -67.8906) -> (109.8601, -68.7585)
  line L3358 (109.8601, -68.7585) -> (109.8582, -68.7681)
  line L3359 (109.8582, -68.7681) -> (109.8446, -68.7816)
  line L3360 (109.8446, -68.7816) -> (109.8351, -68.7835)
  line L3361 (109.8351, -68.7835) -> (107.1812, -68.7835)
  line L3362 (107.1812, -68.7835) -> (107.1812, -72.6281)
  line L3363 (107.1812, -72.6281) -> (107.1812, -73.8187)
  line L3364 (107.1812, -73.8187) -> (107.1793, -73.8283)
  line L3365 (107.1793, -73.8283) -> (107.1657, -73.8418)
  line L3366 (107.1657, -73.8418) -> (107.1562, -73.8437)
  line L3367 (107.1562, -73.8437) -> (102.6913, -73.8437)
  line L3368 (102.6913, -73.8437) -> (102.3937, -73.8437)
  line L3369 (102.3937, -73.8437) -> (102.3841, -73.8418)
  line L3370 (102.3841, -73.8418) -> (102.3706, -73.8283)
  line L3371 (102.3706, -73.8283) -> (102.3687, -73.8187)
  line L3372 (102.3687, -73.8187) -> (102.3687, -70.8671)
  line L3373 (102.3687, -70.8671) -> (100.9304, -70.8671)
  line L3374 (100.9304, -70.8671) -> (100.9304, -72.6281)
  line L3375 (100.9304, -72.6281) -> (100.9285, -72.6376)
  line L3376 (100.9285, -72.6376) -> (100.915, -72.6512)
  line L3377 (100.915, -72.6512) -> (100.9054, -72.6531)
  line L3378 (100.9054, -72.6531) -> (98.5241, -72.6531)
  line L3379 (98.5241, -72.6531) -> (98.5146, -72.6512)
  line L3380 (98.5146, -72.6512) -> (98.501, -72.6376)
  line L3381 (98.501, -72.6376) -> (98.4991, -72.6281)
  line L3382 (98.4991, -72.6281) -> (98.4991, -70.5695)
  line L3383 (98.4991, -70.5695) -> (96.1429, -70.5695)
  line L3384 (96.1429, -70.5695) -> (96.1333, -70.5676)
  line L3385 (96.1333, -70.5676) -> (96.1198, -70.554)
  line L3386 (96.1198, -70.554) -> (96.1179, -70.5445)
  line L3387 (96.1179, -70.5445) -> (96.1179, -67.2703)
  line L3388 (96.1179, -67.2703) -> (96.1198, -67.2607)
  line L3389 (96.1198, -67.2607) -> (96.1333, -67.2472)
  line L3390 (96.1333, -67.2472) -> (96.1429, -67.2453)
  line L3391 (96.1429, -67.2453) -> (98.4991, -67.2453)
  line L3392 (98.4991, -67.2453) -> (98.4991, -64.2937)
  line L3393 (98.4991, -64.2937) -> (98.501, -64.2841)
  line L3394 (98.501, -64.2841) -> (98.5146, -64.2706)
  line L3395 (98.5146, -64.2706) -> (98.5241, -64.2687)
  line L3396 (98.5241, -64.2687) -> (112.2163, -64.2687)
  line L3397 (112.2163, -64.2687) -> (112.2259, -64.2706)
  line L3398 (98.5491, -64.3187) -> (98.5491, -67.2703)
  line L3399 (98.5491, -67.2703) -> (98.5472, -67.2798)
  line L3400 (98.5472, -67.2798) -> (98.5337, -67.2934)
  line L3401 (98.5337, -67.2934) -> (98.5241, -67.2953)
  line L3402 (98.5241, -67.2953) -> (96.1679, -67.2953)
  line L3403 (96.1679, -67.2953) -> (96.1679, -70.5195)
  line L3404 (96.1679, -70.5195) -> (98.5241, -70.5195)
  line L3405 (98.5241, -70.5195) -> (98.5337, -70.5214)
  line L3406 (98.5337, -70.5214) -> (98.5472, -70.5349)
  line L3407 (98.5472, -70.5349) -> (98.5491, -70.5445)
  line L3408 (98.5491, -70.5445) -> (98.5491, -72.6031)
  line L3409 (98.5491, -72.6031) -> (100.8804, -72.6031)
  line L3410 (100.8804, -72.6031) -> (100.8804, -70.8421)
  line L3411 (100.8804, -70.8421) -> (100.8823, -70.8326)
  line L3412 (100.8823, -70.8326) -> (100.8958, -70.819)
  line L3413 (100.8958, -70.819) -> (100.9054, -70.8171)
  line L3414 (100.9054, -70.8171) -> (102.3937, -70.8171)
  line L3415 (102.3937, -70.8171) -> (102.4032, -70.819)
  line L3416 (102.4032, -70.819) -> (102.4168, -70.8326)
  line L3417 (102.4168, -70.8326) -> (102.4187, -70.8421)
  line L3418 (102.4187, -70.8421) -> (102.4187, -73.7937)
  line L3419 (102.4187, -73.7937) -> (102.6913, -73.7937)
  line L3420 (102.6913, -73.7937) -> (107.1312, -73.7937)
  line L3421 (107.1312, -73.7937) -> (107.1312, -72.6281)
  line L3422 (107.1312, -72.6281) -> (107.1312, -68.7585)
  line L3423 (107.1312, -68.7585) -> (107.1331, -68.749)
  line L3424 (107.1331, -68.749) -> (107.1466, -68.7354)
  line L3425 (107.1466, -68.7354) -> (107.1562, -68.7335)
  line L3426 (107.1562, -68.7335) -> (109.8101, -68.7335)
  line L3427 (109.8101, -68.7335) -> (109.8101, -67.8656)
  line L3428 (109.8101, -67.8656) -> (109.812, -67.856)
  line L3429 (109.812, -67.856) -> (109.8255, -67.8425)
  line L3430 (109.8255, -67.8425) -> (109.8351, -67.8406)
  line L3431 (109.8351, -67.8406) -> (112.1913, -67.8406)
  line L3432 (112.1913, -67.8406) -> (112.1913, -64.3187)
  line L3433 (112.1913, -64.3187) -> (98.5491, -64.3187)
  line L3434 (131.2758, -64.2705) -> (131.2894, -64.2841)
  line L3435 (131.2894, -64.2841) -> (131.2913, -64.2936)
  line L3436 (131.2913, -64.2936) -> (131.2913, -67.8655)
  line L3437 (131.2913, -67.8655) -> (131.2894, -67.8751)
  line L3438 (131.2894, -67.8751) -> (131.2758, -67.8886)
  line L3439 (131.2758, -67.8886) -> (131.2663, -67.8905)
  line L3440 (131.2663, -67.8905) -> (128.91, -67.8905)
  line L3441 (128.91, -67.8905) -> (128.91, -68.7585)
  line L3442 (128.91, -68.7585) -> (128.9081, -68.768)
  line L3443 (128.9081, -68.768) -> (128.8946, -68.7816)
  line L3444 (128.8946, -68.7816) -> (128.885, -68.7835)
  line L3445 (128.885, -68.7835) -> (126.2311, -68.7835)
  line L3446 (126.2311, -68.7835) -> (126.2311, -72.628)
  line L3447 (126.2311, -72.628) -> (126.2311, -73.8186)
  line L3448 (126.2311, -73.8186) -> (126.2292, -73.8282)
  line L3449 (126.2292, -73.8282) -> (126.2157, -73.8417)
  line L3450 (126.2157, -73.8417) -> (126.2061, -73.8436)
  line L3451 (126.2061, -73.8436) -> (121.7413, -73.8436)
  line L3452 (121.7413, -73.8436) -> (121.4436, -73.8436)
  line L3453 (121.4436, -73.8436) -> (121.434, -73.8417)
  line L3454 (121.434, -73.8417) -> (121.4205, -73.8282)
  line L3455 (121.4205, -73.8282) -> (121.4186, -73.8186)
  line L3456 (121.4186, -73.8186) -> (121.4186, -70.8671)
  line L3457 (121.4186, -70.8671) -> (119.9803, -70.8671)
  line L3458 (119.9803, -70.8671) -> (119.9803, -72.628)
  line L3459 (119.9803, -72.628) -> (119.9784, -72.6376)
  line L3460 (119.9784, -72.6376) -> (119.9649, -72.6511)
  line L3461 (119.9649, -72.6511) -> (119.9553, -72.653)
  line L3462 (119.9553, -72.653) -> (117.5741, -72.653)
  line L3463 (117.5741, -72.653) -> (117.5645, -72.6511)
  line L3464 (117.5645, -72.6511) -> (117.551, -72.6376)
  line L3465 (117.551, -72.6376) -> (117.5491, -72.628)
  line L3466 (117.5491, -72.628) -> (117.5491, -70.5694)
  line L3467 (117.5491, -70.5694) -> (115.1928, -70.5694)
  line L3468 (115.1928, -70.5694) -> (115.1833, -70.5675)
  line L3469 (115.1833, -70.5675) -> (115.1697, -70.554)
  line L3470 (115.1697, -70.554) -> (115.1678, -70.5444)
  line L3471 (115.1678, -70.5444) -> (115.1678, -67.2702)
  line L3472 (115.1678, -67.2702) -> (115.1697, -67.2606)
  line L3473 (115.1697, -67.2606) -> (115.1833, -67.2471)
  line L3474 (115.1833, -67.2471) -> (115.1928, -67.2452)